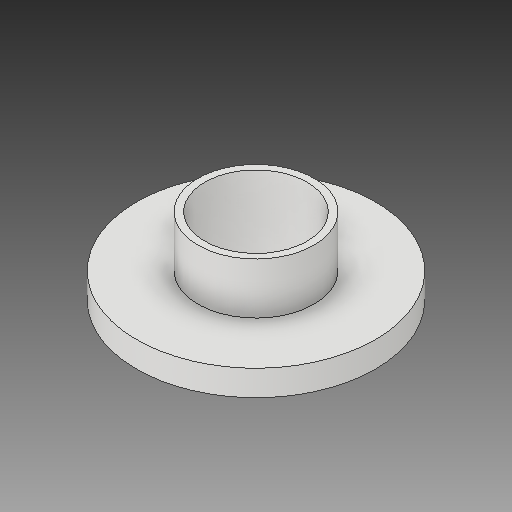
# Autodesk Inventor part: D6068-4530
Saved by Autodesk Inventor 2018 (Build 220112000, 112)
## iProperties
Created: 2016-08-26
Part Number: D6068-4530
Material: アセタール樹脂、白
Document SubType Name: Modeling
Designer: hiro
Density: 1.425 g/cm^3
Appearance: 滑らか - 白
Mass: 0.302988 g
Surface Area: 4.66212 cm^2
Volume: 0.212623 cm^3
Author: hiro
Autodesk Inventor part; units mm, degrees
ref_plane "YZ Plane" through (0, 0, 0) normal (1, 0, 0) x (0, 1, 0)
ref_plane "XZ Plane" through (0, 0, 0) normal (0, 1, 0) x (-1, 0, 0)
ref_plane "XY Plane" through (0, 0, 0) normal (0, 0, 1) x (1, 0, 0)
sketch "スケッチ1" plane through (0, 0, 0) normal (0, 0, 1) x (1, 0, 0)
  line L0 (3, 2.25) -> (3, -2.25)
  line L1 (3, -2.25) -> (7, -2.25)
  line L2 (7, -2.25) -> (7, -0.75)
  line L3 (7, -0.75) -> (3.4, -0.75)
  line L4 (3.4, -0.75) -> (3.4, 2.25)
  line L5 (3.4, 2.25) -> (3, 2.25)
  line L6 (0, 0) -> (0, 3.1564) construction
  point P0 (3, 0)
  dimension "d0" = 6
  dimension "d1" = 6.8
  dimension "d2" = 14
  dimension "d3" = 1.5
  dimension "d4" = 3
  constraints: 14 end point, 4 perpendicular, 2 vertical, 1 horizontal, 1 horizontal alignment, 1 midpoint
  measures "d0" diameter of L0 L6
  measures "d1" diameter of L4 L6
  measures "d2" diameter of L2 L6
  measures "d3" distance of L1.end L2.end
  measures "d4" distance of L3.end L4.end
revolve "回転1" add sketch "スケッチ1" angle 360 about axis through (0, 0, 0) along (0, 1, 0)
